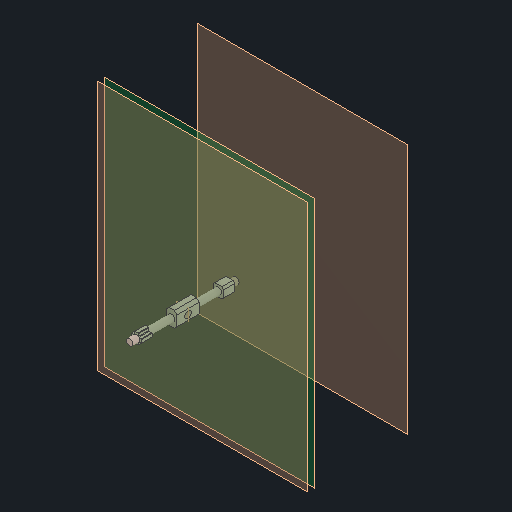
# Autodesk Inventor part: EjeEngraneGrua
Saved by Autodesk Inventor 2026.2 (Build 302298010, 298A)
## iProperties
Created: 2026-04-22
Part Number: EjeEngraneGrua
Material: Genérico
Document SubType Name: Modeling
Designer: Jose Carlos
Density: 1 g/cm^3
Appearance: Valor por defecto
Author: Jose Carlos
Autodesk Inventor part; units mm, degrees
ref_plane "YZ Plane" through (0, 0, 0) normal (1, 0, 0) x (0, 1, 0)
ref_plane "XZ Plane" through (0, 0, 0) normal (0, 1, 0) x (-1, 0, 0)
ref_plane "XY Plane" through (0, 0, 0) normal (0, 0, 1) x (1, 0, 0)
ref_plane "Plano de trabajo1" through (0, 0, 0) normal (0, 0, 1) x (1, 0, 0)
sketch "Boceto1" plane through (0, 0, 0) normal (0, 0, 1) x (1, 0, 0)
  circle A0 centre (-34.5, -38.2272) radius 1.45
  point P0 (0, 0)
  dimension "d0" = 2.9
  constraints: 1 centre point, 1 coincident, 1 other
  measures "d0" diameter of A0
ref_plane "Plano de trabajo2" through (-44.5, -51.5, -48) normal (0, 0, -1) x (0, 1, 0)
extrude "Extrusión1" add sketch "Boceto1" against normal up to surface (48 mm away)
ref_plane "Plano de trabajo3" through (0, 0, -45.1) normal (0, 0, 1) x (1, 0, 0)
sketch "Boceto2" plane through (0, 0, -45.1) normal (0, 0, 1) x (1, 0, 0)
  line L0 (-32.1, -35.8272) -> (-36.9, -35.8272)
  line L1 (-36.9, -35.8272) -> (-36.9, -40.6272)
  line L2 (-36.9, -40.6272) -> (-32.1, -40.6272)
  line L3 (-32.1, -40.6272) -> (-32.1, -35.8272)
  line L4 (-32.1, -35.8272) -> (-36.9, -40.6272) construction
  line L5 (-36.9, -35.8272) -> (-32.1, -40.6272) construction
  point P0 (0, 0)
  point P1 (-34.5, -38.2272)
  dimension "d3" = 4.8
  dimension "d4" = 4.8
  constraints: 12 end point, 2 midpoint, 2 parallel, 1 horizontal, 1 perpendicular, 1 other
  measures "d3" distance of L1.end L2.end
  measures "d4" distance of L0.end L1.end
extrude "Extrusión2" add sketch "Boceto2" along normal blind 5
chamfer "Chaflán1" distance 0.8 angle 45 4 edges at (-36.9, -40.6272, -42.6) (-36.9, -35.8272, -42.6) (-32.1, -35.8272, -42.6) (-32.1, -40.6272, -42.6)
ref_plane "Plano de trabajo4" through (0, 0, -3.1) normal (0, 0, -1) x (-1, 0, 0)
sketch "Boceto3" plane through (0, 0, -3.1) normal (0, 0, -1) x (-1, 0, 0)
  line L0 (32.1, -39.1272) -> (36.9, -39.1272)
  line L1 (36.9, -39.1272) -> (36.9, -37.3272)
  line L2 (36.9, -37.3272) -> (32.1, -37.3272)
  line L3 (32.1, -37.3272) -> (32.1, -39.1272)
  line L4 (32.1, -39.1272) -> (36.9, -37.3272) construction
  line L5 (36.9, -39.1272) -> (32.1, -37.3272) construction
  line L6 (33.6, -40.6272) -> (35.4, -40.6272)
  line L7 (35.4, -40.6272) -> (35.4, -35.8272)
  line L8 (35.4, -35.8272) -> (33.6, -35.8272)
  line L9 (33.6, -35.8272) -> (33.6, -40.6272)
  line L10 (33.6, -40.6272) -> (35.4, -35.8272) construction
  line L11 (35.4, -40.6272) -> (33.6, -35.8272) construction
  circle A0 centre (34.5, -38.2272) radius 1.4
  point P0 (0, 0)
  point P1 (35.5724, -37.3272)
  point P2 (35.4, -37.1548)
  point P3 (33.6, -37.1548)
  point P4 (33.4276, -37.3272)
  point P5 (33.4276, -39.1272)
  point P6 (33.6, -39.2996)
  point P7 (35.4, -39.2996)
  point P8 (35.5724, -39.1272)
  dimension "d12" = 1.8
  dimension "d13" = 4.8
  dimension "d14" = 2.8
  constraints: 24 end point, 4 midpoint, 4 parallel, 4 perpendicular, 2 horizontal, 1 centre point, 1 coincident, 1 other
  measures "d12" distance of L0.end L1.end
  measures "d13" distance of L1.end L2.end
  measures "d14" diameter of A0
ref_plane "Plano de trabajo5" through (-39.1917, -42.9189, -7.7627) normal (0, 0, -1) x (0, 1, 0)
extrude "Extrusión3" add sketch "Boceto3" along normal up to surface (4.6627 mm away)
chamfer "Chaflán2" distance 0.2 angle 45 8 edges at (-35.4, -35.8272, -5.4314) (-36.9, -37.3272, -5.4314) (-36.9, -39.1272, -5.4314) (-35.4, -40.6272, -5.4314) (-33.6, -40.6272, -5.4314) (-33.6, -35.8272, -5.4314) (-32.1, -37.3272, -5.4314) (-32.1, -39.1272, -5.4314)
ref_plane "Plano de trabajo6" through (-34.5, -38.2272, -24) normal (0, 0, 1) x (1, 0, 0)
sketch "Boceto4" plane through (-34.5, -38.2272, -24) normal (0, 0, 1) x (1, 0, 0)
  circle A0 centre (0, 0) radius 1.55 construction
  line L0 (2.4, 3.5) -> (-2.4, 3.5)
  line L1 (-2.4, 3.5) -> (-2.4, -3.5)
  line L2 (-2.4, -3.5) -> (2.4, -3.5)
  line L3 (2.4, -3.5) -> (2.4, 3.5)
  line L4 (2.4, 3.5) -> (-2.4, -3.5) construction
  line L5 (-2.4, 3.5) -> (2.4, -3.5) construction
  point P0 (34.5, 38.2272)
  dimension "d20" = 7
  dimension "d26" = 4.8
  constraints: 12 end point, 2 midpoint, 2 parallel, 1 horizontal, 1 perpendicular
  measures "d20" distance of L0.end L1.end
  measures "d26" distance of L0.start L0.end
extrude "Extrusión4" add sketch "Boceto4" along normal mid plane 10
chamfer "Chaflán3" distance 1.2 angle 45 4 edges at (-36.9, -34.7272, -24) (-36.9, -41.7272, -24) (-32.1, -34.7272, -24) (-32.1, -41.7272, -24)
sketch "Boceto5" plane through (-36.9, -40.5272, -19) normal (-1, 0, 0) x (0, 0, 1)
  line L0 (-5, 48.8726) -> (-5, -9.5454) construction
  line L1 (-5, 2.3) -> (-5, -1.2) construction
  line L2 (-10, -1.2) -> (0, -1.2) construction
  line L3 (-5, 2.3) -> (-5, 5.8) construction
  line L4 (-10, 5.8) -> (0, 5.8) construction
  point P0 (19, 40.5272)
  constraints: 4 end point, 2 midpoint, 1 collinear, 1 point on line
hole "Agujero1" at (-36.9, -38.2272, -24) direction (1, 0, 0) diameter 3 end through all
